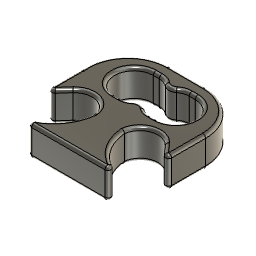
boat_hook (Autodesk Fusion 360 design; units mm, degrees)
Autodesk Fusion 360 part; units mm, degrees
sketch "Sketch1" plane through (0, 0, 0) normal (0, 0, 1) x (1, 0, 0)
  line L0 (0, 0) -> (26, 0)
  line L1 (26, 0) -> (26, 13)
  line L2 (26, 13) -> (0, 13)
  line L3 (0, 13) -> (0, 0)
  line L4 (-5, -5) -> (31, -5)
  line L5 (31, -5) -> (31, 18)
  line L6 (31, 18) -> (-5, 18)
  line L7 (-5, 18) -> (-5, -5)
  line L8 (-5, 0) -> (-10, 0)
  line L9 (-10, 0) -> (-10, -15)
  line L10 (-10, -15) -> (-5, -15)
  line L11 (-5, -15) -> (-5, 0)
  line L12 (31, 0) -> (36, 0)
  line L13 (36, 0) -> (36, -15)
  line L14 (36, -15) -> (31, -15)
  line L15 (31, -15) -> (31, 0)
  line L16 (7, -5) -> (19, -5)
  line L17 (19, -5) -> (19, -27)
  line L18 (19, -27) -> (7, -27)
  line L19 (7, -27) -> (7, -5)
  dimension "d1" = 26
  dimension "d2" = 13
  dimension "d3" = 36
  dimension "d4" = 12
  dimension "d5" = 22
  constraint horizontal L0
  constraint vertical L1
  constraint horizontal L2
  constraint vertical L3
  constraint coincident L0.start L3.end
  constraint horizontal L4
  constraint vertical L5
  constraint horizontal L6
  constraint vertical L7
  constraint horizontal L8
  constraint vertical L9
  constraint horizontal L10
  constraint vertical L11
  constraint coincident L7 L8.start
  constraint horizontal L12
  constraint vertical L13
  constraint horizontal L14
  constraint vertical L15
  constraint coincident L5 L12.start
  constraint horizontal L16
  constraint vertical L17
  constraint horizontal L18
  constraint vertical L19
  constraint coincident L4 L16.start
  measures "d1" distance of L0.start L0.end
  measures "d2" distance of L0.start L2.end
  measures "d3" distance of L4.start L4.end
  measures "d4" distance of L16.start L16.end
  measures "d5" distance of L16.start L18.end
sketch "Sketch2" plane through (0, 0, 0) normal (0, 0, 1) x (1, 0, 0)
  line L0 (45, 0) -> (85, 0)
  line L1 (85, 12) -> (85, 30)
  line L2 (71.0033, 40) -> (58.9967, 40)
  line L3 (45, 30) -> (45, 12)
  line L4 (45, 29) -> (45, 30)
  line L5 (85, 29) -> (85, 30)
  arc A0 (72, 22.5) -> (72, 35.5) centre (72, 29) ccw
  arc A1 (58, 35.5) -> (58, 22.5) centre (58, 29) ccw
  arc A2 (84.9642, 25) -> (70.9967, 40) centre (71, 26) ccw
  arc A3 (59.0033, 40) -> (45.0358, 25) centre (59, 26) ccw
  line L6 (45, 25) -> (45.0358, 25)
  line L7 (77.1235, 25) -> (77, 25)
  line L8 (45, 0) -> (48, 0)
  line L9 (48, 12) -> (45, 12)
  line L10 (45, 12) -> (49.5525, 17.0274)
  line L11 (85, 12) -> (80.4475, 17.0274)
  arc A4 (45.5803, 29.9888) -> (45, 30) centre (45, 15) ccw
  arc A5 (45, 0) -> (59.9498, 13.7743) centre (45, 15) ccw
  arc A6 (85, 30) -> (84.4198, 29.9888) centre (85, 15) ccw
  arc A7 (70.0502, 13.7743) -> (85, 0) centre (85, 15) ccw
  arc A8 (80.4475, 17.0274) -> (70.0502, 13.7743) centre (76, 13) ccw
  arc A9 (59.9498, 13.7743) -> (49.5525, 17.0274) centre (54, 13) ccw
  arc A10 (65, 30.5) -> (60, 35.5) centre (60, 30.5) ccw
  arc A11 (60, 22.5) -> (65, 27.5) centre (60, 27.5) ccw
  arc A12 (65, 27.5) -> (70, 22.5) centre (70, 27.5) ccw
  arc A13 (70, 35.5) -> (65, 30.5) centre (70, 30.5) ccw
  line L12 (58, 22.5) -> (60, 22.5)
  line L13 (70, 22.5) -> (72, 22.5)
  line L14 (58, 35.5) -> (60, 35.5)
  line L15 (70, 35.5) -> (72, 35.5)
  dimension "d6" = 40
  dimension "d10" = 13
  dimension "d13" = 13
  dimension "d15" = 28
  dimension "d16" = 12
  dimension "d17" = 3
  dimension "d18" = 12
  dimension "d19" = 12
  dimension "d22" = 5
  dimension "d24" = 10
  dimension "d25" = 5
  constraint horizontal L0
  constraint vertical L1
  constraint horizontal L2
  constraint vertical L3
  constraint vertical L4
  constraint vertical L5
  constraint tangent A0 L12
  constraint coincident L2 A3.start
  constraint coincident L2 A2.end
  constraint coincident L3 L6.start
  constraint perpendicular L3 L6
  constraint perpendicular L1 L7
  constraint horizontal L8
  constraint horizontal L9
  constraint coincident L3 A4.centre
  constraint coincident L1 A6.centre
  constraint tangent L10 A9
  constraint tangent L11 A8
  constraint coincident A3 A4.start
  constraint concentric A4 A5
  constraint concentric A6 A7
  constraint coincident A2 A6.end
  constraint coincident A2 L2.start
  constraint coincident A3 L2.end
  constraint coincident A0 L7.start
  constraint collinear L12 L13
  constraint collinear L14 L15
  measures "d6" distance of L0.start L0.end
  measures "d10" diameter of A1
  measures "d13" diameter of A0
  measures "d15" diameter of A3
  measures "d16" diameter of A9
  measures "d17" distance of L0.start L8.end
  measures "d18" distance of L0.start L3.end
  measures "d19" diameter of A8
  measures "d22" distance of A10.start A13.centre
  measures "d24" distance of A11.start A12.end
  measures "d25" distance of A11.start A11.centre
sketch "Sketch3" plane through (0, 0, 0) normal (0, 0, 1) x (1, 0, 0)
  line L0 (105, 0) -> (150, 0)
  line L1 (150, 11.5) -> (150, 31)
  line L2 (136, 45) -> (119, 45)
  line L3 (105, 32.5) -> (105, 11.5)
  line L4 (119, 45) -> (136, 45)
  line L5 (150, 31) -> (150, 20)
  line L6 (105, 20) -> (105, 32.5)
  line L7 (119, 45) -> (127.5, 45)
  line L8 (105.0806, 32.5) -> (105, 32.5)
  arc A0 (119, 45) -> (105, 31) centre (119, 31) ccw
  line L9 (136, 41) -> (119, 41)
  line L10 (136, 24) -> (119, 24)
  arc A1 (119, 41) -> (119.0041, 24) centre (119, 32.5) ccw
  arc A2 (135.9975, 24) -> (136, 41) centre (136, 32.5) ccw
  arc A3 (127.3397, 20) -> (127.5, 19.8757) centre (136, 31) ccw
  arc A4 (150, 31) -> (136, 45) centre (136, 31) ccw
  line L11 (105, 0) -> (115.9939, 3.3741)
  line L12 (150, 0) -> (139.0061, 3.3741)
  arc A5 (115.9939, 3.3741) -> (105, 11.5) centre (113.5, 11.5) ccw
  arc A6 (150, 11.5) -> (139.0061, 3.3741) centre (141.5, 11.5) ccw
  dimension "d26" = 45
  dimension "d33" = 17
  dimension "d34" = 17
  dimension "d36" = 14
  dimension "d37" = 8.5
  dimension "d38" = 8.5
  constraint horizontal L0
  constraint vertical L1
  constraint horizontal L2
  constraint vertical L3
  constraint horizontal L4
  constraint vertical L5
  constraint vertical L6
  constraint horizontal L7
  constraint horizontal L8
  constraint tangent L2 A3
  constraint tangent L5 A3
  constraint coincident L3 A0.end
  constraint horizontal L9
  constraint horizontal L10
  constraint coincident L10.start A2
  constraint coincident L10 A2.start
  constraint coincident L10 A1.end
  constraint concentric A3 A4
  constraint coincident A0 L8.start
  constraint tangent L3 A5
  constraint tangent L1 A6
  constraint tangent L11 A5
  constraint tangent L12 A6
  measures "d26" distance of L0.start L0.end
  measures "d33" diameter of A1
  measures "d34" diameter of A2
  measures "d36" radius of A3
  measures "d37" radius of A5
  measures "d38" radius of A6
extrude "Extrude1" add sketch "Sketch2" along normal blind 10 contours L0 L1 L2 L3 A2 A3 L6 L8 L10 L11 A5 A7 A8 A9
fillet "Fillet1" radius 3 2 edges at (65, 30.5, 5) (65, 27.5, 5)
fillet "Fillet2" radius 1 2 edges at (85, 0, 5) (45, 0, 5)
fillet "Fillet3" radius 1 2 edges at (85, 12, 5) (45, 12, 5)
fillet "Fillet4" radius 1 2 faces at (65.8096, 18.0128, 10) (65.8096, 18.0128, 0)
scale "Scale1" factor 1.36 about (66.875, 23.5969, 9) bodies 1
